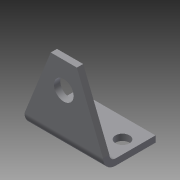
# Autodesk Inventor part: arm assembly mount plate
Saved by Autodesk Inventor 2013 (Build 170138000, 138)
## iProperties
Created: 2013-01-20
Part Number: arm assembly mount plate
Material: Generic
Document SubType Name: Sheet Metal
Designer: Arpan
Density: 1 g/cm^3
Sheet Metal Rule: Default
Mass: 5.09807 g
Surface Area: 40.9054 cm^2
Volume: 5.09807 cm^3
Author: Arpan
Autodesk Inventor part; units mm, degrees
ref_plane "YZ Plane" through (0, 0, 0) normal (1, 0, 0) x (0, 1, 0)
ref_plane "XZ Plane" through (0, 0, 0) normal (0, 1, 0) x (-1, 0, 0)
ref_plane "XY Plane" through (0, 0, 0) normal (0, 0, 1) x (1, 0, 0)
sketch "Sketch1" plane through (0, 0, 0) normal (0, 0, 1) x (1, 0, 0)
  line L0 (0, 0) -> (-12.7, 0)
  line L1 (-6.35, 0) -> (-6.35, -31.75)
  line L2 (-6.35, -31.75) -> (-25.4, -31.75)
  line L3 (-25.4, -31.75) -> (-12.7, 0)
  line L4 (-6.35, -31.75) -> (12.7, -31.75)
  line L5 (0, 0) -> (12.7, -31.75)
  dimension "d0" = 12.7
  dimension "d1" = 31.75
  dimension "d2" = 19.05
  dimension "d3" = 19.05
  measures "d0" distance of L0.start L0.end
  measures "d1" distance of L1.start L1.end
  measures "d2" distance of L1.end L2.end
  measures "d3" distance of L1.end L4.end
extrude "Plate1" add sketch "Sketch1" along normal blind 3.048
sketch "Sketch2" plane through (0, 0, 3.048) normal (0, 0, 1) x (1, 0, 0)
  line L0 (-12.7, 0) -> (0, 0) projected
  line L1 (12.7, -31.75) -> (-25.4, -31.75) projected
  line L2 (-6.35, 0) -> (-6.35, -12.7)
  circle A0 centre (-6.35, -12.7) radius 4.7625
  dimension "d7" = 12.7
  dimension "d8" = 9.525
  constraints: 2 end point, 1 centre point, 1 coincident, 1 midpoint, 1 perpendicular
  measures "d7" distance of L2.start L2.end
  measures "d8" diameter of A0
extrude "Cut1" cut sketch "Sketch2" against normal blind 3.048
sketch "Sketch3" plane through (-25.4, -34.798, -3.048) normal (0, -1, 0) x (1, 0, 0)
  line L0 (38.1, 0) -> (0, 0)
  line L1 (0, 0) -> (0, -19.304)
  line L2 (0, -19.304) -> (38.1, -19.304)
  line L3 (38.1, -19.304) -> (38.1, 0)
  constraints: 6 end point, 1 horizontal, 1 perpendicular, 1 vertical
edge flange "Flange1" height 25.4 angle 90 thickness 3.048 bend radius 3.048 thickness toward (0, -1, 0) relief tear relief width 3.048 relief depth 1.524 edges at (-6.35, -31.75, 0) wall of the first edge with corners at (12.7, -34.798, -3.048) (-25.4, -34.798, -3.048) (-25.4, -34.798, -22.352) (12.7, -34.798, -22.352)
bend "Bend1"
corner "Corner1"
sketch "Sketch4" plane through (-25.4, -34.798, -22.352) normal (0, 1, 0) x (1, 0, 0)
  line L0 (38.1, 0) -> (38.1, -19.304) projected
  line L1 (0, 0) -> (0, -19.304) projected
  line L2 (0, -9.652) -> (6.35, -9.652)
  circle A0 centre (6.35, -9.652) radius 3.3782
  line L3 (38.1, -9.652) -> (31.75, -9.652)
  circle A1 centre (31.75, -9.652) radius 3.3782
  point P0 (25.4, -22.352)
  dimension "d21" = 6.35
  dimension "d23" = 6.7564
  dimension "d24" = 6.35
  dimension "d25" = 6.7564
  constraints: 4 end point, 2 centre point, 2 coincident, 2 midpoint, 1 collinear, 1 perpendicular
  measures "d21" distance of L2.start L2.end
  measures "d23" diameter of A0
  measures "d24" distance of L3.start L3.end
  measures "d25" diameter of A1
extrude "Cut2" cut sketch "Sketch4" against normal blind 3.048
equation "\"d9\" = Thickness"
equation "\"d26\" = Thickness"
equation "\"d11\" = BendReliefWidth"
equation "\"d12\" = BendReliefDepth"
equation "\"d13\" = MinimumRemnant"
equation "\"d14\" = BendRadius"
equation "\"d17\" = BendRadius"
equation "\"d18\" = CornerReliefSize"
equation "\"d19\" = GapSize"
equation "\"d20\" = JacobiRadiusSize"
equation "\"BendRadius\" = Thickness"
equation "\"BendReliefWidth\" = Thickness"
equation "\"BendReliefDepth\" = 0.5 * Thickness"
equation "\"CornerReliefSize\" = 4 * Thickness"
equation "\"MinimumRemnant\" = 2 * Thickness"
equation "\"TransitionRadius\" = BendRadius"
equation "\"JacobiRadiusSize\" = Thickness"
equation "\"GapSize\" = Thickness"
equation "\"d4\" = BendRadius"
equation "\"Thickness\" = 3.048"
body "Solid1"
